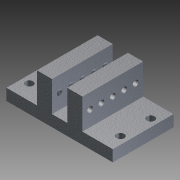
# Autodesk Inventor part: solid_alum_chain_grabber
Saved by Autodesk Inventor 2011 (Build 150239000, 239)
## iProperties
Created: 2013-01-17
Part Number: solid_alum_chain_grabber
Document SubType Name: Modeling
Designer: Christopher
Density: 1 g/cm^3
Author: Christopher
Autodesk Inventor part; units mm, degrees
ref_plane "YZ Plane" through (0, 0, 0) normal (1, 0, 0) x (0, 1, 0)
ref_plane "XZ Plane" through (0, 0, 0) normal (0, 1, 0) x (-1, 0, 0)
ref_plane "XY Plane" through (0, 0, 0) normal (0, 0, 1) x (1, 0, 0)
sketch "Sketch1" plane through (0, 0, 0) normal (0, 0, 1) x (1, 0, 0)
  line L0 (-12.1705, 0) -> (76.7295, 0)
  line L1 (76.7295, 0) -> (76.7295, 9.525)
  line L2 (76.7295, 9.525) -> (51.3295, 9.525)
  line L3 (-12.1705, 0) -> (-12.1705, 9.525)
  line L4 (-12.1705, 9.525) -> (13.2295, 9.525)
  line L5 (13.2295, 9.525) -> (13.2295, 34.925)
  line L6 (51.3295, 9.525) -> (51.3295, 34.925)
  line L7 (13.2295, 34.925) -> (25.9295, 34.925)
  line L8 (25.9295, 34.925) -> (25.9295, 9.525)
  line L9 (25.9295, 9.525) -> (38.6295, 9.525)
  line L10 (38.6295, 9.525) -> (38.6295, 34.925)
  line L11 (38.6295, 34.925) -> (51.3295, 34.925)
  point P0 (0, 0)
  dimension "d0" = 88.9
  dimension "d1" = 9.525
  dimension "d2" = 25.4
  dimension "d3" = 25.4
  dimension "d4" = 25.4
  dimension "d8" = 12.7
  dimension "d9" = 12.7
  constraints: 24 end point, 5 parallel, 5 perpendicular, 1 collinear, 1 horizontal
  measures "d0" distance of L0.start L0.end
  measures "d1" distance of L0.end L1.end
  measures "d2" distance of L1.end L2.end
  measures "d3" distance of L3.end L4.end
  measures "d4" distance of L4.end L5.end
  measures "d8" distance of L8.end L9.end
  measures "d9" distance of L10.end L6.end
extrude "Extrusion1" add sketch "Sketch1" against normal blind 50.8
sketch "Sketch2" plane through (51.3295, 9.525, 0) normal (0, 1, 0) x (1, 0, 0)
  line L0 (25.4, 50.8) -> (0, 50.8) projected
  line L1 (25.4, 0) -> (25.4, 50.8) projected
  line L2 (-63.5, 0) -> (-63.5, 50.8) projected
  point P0 (-51.3295, 0)
  point P1 (19.05, 12.7)
  point P2 (19.05, 38.1)
  point P3 (-57.15, 38.1)
  point P4 (-57.15, 12.7)
  dimension "d12" = 6.35
  dimension "d13" = 6.35
  dimension "d14" = 25.4
  dimension "d15" = 12.7
  constraints: 2 horizontal alignment, 2 vertical alignment
  measures "d12" distance from line of L2 point (-57.15, 12.7)
  measures "d13" distance from line of L1 point (19.05, 12.7)
  measures "d14" distance of point (19.05, 38.1) point (19.05, 12.7)
  measures "d15" distance from line of L0 point (19.05, 38.1)
sketch "Sketch3" plane through (51.3295, 9.525, 0) normal (1, 0, 0) x (0, 0, -1)
  line L0 (0, 25.4) -> (50.8, 25.4) projected
  line L1 (0, 0) -> (0, 25.4) projected
  point P0 (0, -9.525)
  point P1 (6.35, 12.7)
  point P2 (15.875, 12.7)
  point P3 (25.4, 12.7)
  point P4 (34.925, 12.7)
  point P5 (44.45, 12.7)
  dimension "d23" = 9.525
  dimension "d24" = 9.525
  dimension "d25" = 9.525
  dimension "d26" = 9.525
  dimension "d27" = 12.7
  dimension "d28" = 6.35
  constraints: 2 horizontal alignment
  measures "d23" distance of point (15.875, 12.7) point (6.35, 12.7)
  measures "d24" distance of point (25.4, 12.7) point (15.875, 12.7)
  measures "d25" distance of point (34.925, 12.7) point (25.4, 12.7)
  measures "d26" distance of point (34.925, 12.7) point (44.45, 12.7)
  measures "d27" distance from line of L0 point (6.35, 12.7)
  measures "d28" distance from line of L1 point (6.35, 12.7)
hole "Hole1" at (-5.8205, 9.525, -12.7) at (-5.8205, 9.525, -38.1) at (70.3795, 9.525, -38.1) at (70.3795, 9.525, -12.7) direction (0, -1, 0) diameter 6.35 depth 25.4 tip angle 118
hole "Hole2" at (51.3295, 22.225, -6.35) at (51.3295, 22.225, -15.875) at (51.3295, 22.225, -25.4) at (51.3295, 22.225, -34.925) at (51.3295, 22.225, -44.45) direction (-1, 0, 0) diameter 4.7625 depth 25.4 tip angle 118
body "Solid1"
